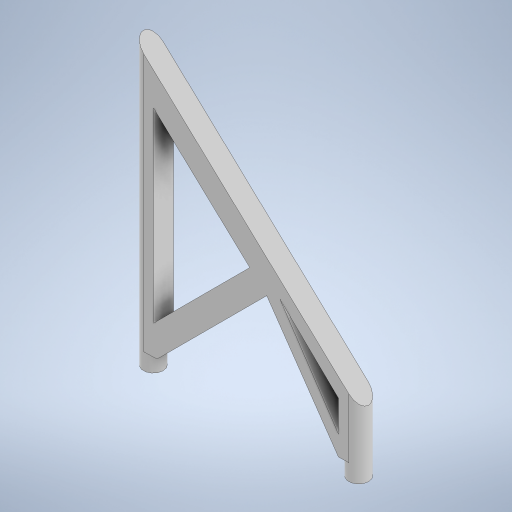
# Autodesk Inventor part: ControlPanel_Middle
Saved by Autodesk Inventor 2024 (Build 280153000, 153)
## iProperties
Created: 2024-04-17
Part Number: ControlPanel_Middle
Material: Generic
Document SubType Name: Modeling
Designer: ringl
Density: 1 g/cm^3
Appearance: Default
Author: ringl
Autodesk Inventor part; units mm, degrees
ref_plane "YZ Plane" through (0, 0, 0) normal (1, 0, 0) x (0, 1, 0)
ref_plane "XZ Plane" through (0, 0, 0) normal (0, 1, 0) x (-1, 0, 0)
sketch "Sketch1" plane through (0, 0, 0) normal (0, 1, 0) x (-1, 0, 0)
  circle A0 centre (0, 0) radius 1.5
  circle A1 centre (0, -51) radius 1.5
  circle A2 centre (30, -1) radius 1.5
  circle A3 centre (30, -50) radius 1.5
  dimension "d0" = 3
  dimension "d1" = 3
  dimension "d2" = 3
  dimension "d3" = 3
  dimension "d5" = 49
  dimension "d6" = 1
  dimension "d7" = 30
  dimension "d8" = 51
  constraints: 4 centre point, 2 vertical alignment, 1 coincident
  measures "d0" diameter of A0
  measures "d1" diameter of A1
  measures "d2" diameter of A2
  measures "d3" diameter of A3
  measures "d5" distance of A3.centre A2.centre
  measures "d6" vertical distance of point (0, 0) A2.centre
  measures "d7" horizontal distance of A2.centre point (0, 0)
  measures "d8" distance of point (0, 0) A1.centre
extrude "Extrusion1" add sketch "Sketch1" along normal blind 2.5
sketch "Sketch2" plane through (-30, 2.5, -1) normal (0, 1, 0) x (1, 0, 0)
  circle A0 centre (0, 0) radius 1.5 projected
  line L0 (0, -1.5) -> (30, -2.5)
  circle A1 centre (30, -1) radius 1.5 projected
  line L1 (30, 0.5) -> (0, 1.5)
  circle A2 centre (0, 49) radius 1.5 projected
  circle A3 centre (30, 50) radius 1.5 projected
  line L2 (0, 50.5) -> (29.95, 51.4992)
  line L3 (30, 48.5) -> (0.05, 47.5008)
  constraints: 8 end point, 8 point on circle, 5 vertical alignment, 2 tangent, 1 parallel
extrude "Extrusion2" add sketch "Sketch2" along normal blind 45
ref_plane "Work Plane1" through (0, 0, 2) normal (0, 0, 1) x (1, 0, 0)
sketch "Sketch3" plane through (0, 0, 2) normal (0, 0, 1) x (1, 0, 0)
  line L0 (1.5, 0) -> (1.5, 47.5) projected
  line L1 (1.5, 10) -> (-31.5, 43)
  line L2 (-31.5, 0) -> (-31.5, 47.5) projected
  line L3 (1.5, 0) -> (-1.5, 0) projected
  line L4 (-31.5, 43) -> (-31.5, 47.5)
  line L5 (-31.5, 0) -> (-31.5, 47.5) projected
  line L6 (1.5, 47.5) -> (1.5, 10)
  line L7 (1.5, 47.5) -> (-31.5, 47.5)
  line L8 (0, 2.5) -> (-29.9001, 2.5) projected
  line L9 (-1.5, 2.5) -> (-28, 2.5)
  line L10 (-28, 2.5) -> (-11.9749, 18.5251)
  line L11 (-11.9749, 18.5251) -> (-1.5, 2.5)
  line L12 (-28.5, 6.9497) -> (-14.4497, 21)
  line L13 (-14.4497, 21) -> (-28.5, 35.0503)
  line L14 (-31.5, 0) -> (-31.5, 47.5) projected
  line L15 (-10.0429, 18.9973) -> (-1.5, 5.5)
  line L16 (-1.5, 5.5) -> (-1.5, 10.1716)
  line L17 (-1.5, 10.1716) -> (-10.0429, 18.9973)
  line L18 (-28.5, 35.0503) -> (-28.5, 6.9497)
  point P0 (0, 0)
  point P1 (-15, 26.5)
  point P2 (-31.5, 38.0503)
  point P3 (-31.5, 3.9497)
  dimension "d14" = 45
  dimension "d15" = 10
  dimension "d18" = 3.5
  dimension "d19" = 3.5
  dimension "d20" = 3.5
  dimension "d21" = 3.5
  dimension "d22" = 45
  dimension "d23" = 3
  dimension "d24" = 1.8
  dimension "d25" = 3
  dimension "d26" = 2
  dimension "d27" = 12.2831
  dimension "d28" = 3
  constraints: 26 end point, 4 point on line, 2 collinear, 2 parallel, 2 vertical, 2 vertical alignment, 1 midpoint, 1 perpendicular
  measures "d14" angle of L3 L1
  measures "d15" distance of L0.start L1.start
  measures "d18" horizontal distance of L2.start L9.end
  measures "d19" distance from line of L1 L10.end
  measures "d20" distance from line of point (-15, 26.5) L13
  measures "d21" distance between parallel lines of L12 L10
  measures "d22" angle of L9 L10
  measures "d23" horizontal distance of L9.start L0.start
  measures "d24" distance from line of L15.start L1
  measures "d25" distance of L9.start L15.end
  measures "d26" distance from line of L1 L16.end
  measures "d27" distance of L16.end L15.start
  measures "d28" distance from line of L5 L12.start
extrude "Extrusion3" cut sketch "Sketch3" against normal through all
sketch "Sketch4" plane through (0, 0, 2) normal (0, 0, 1) x (1, 0, 0)
  line L0 (1.5, 0) -> (-1.5, 0) projected
  line L1 (-31.5, 0) -> (-31.5, 43) projected
  line L2 (1.5, 0) -> (-31.5, 0)
  line L3 (-31.5, 0) -> (-31.5, 43)
  line L4 (-31.5, 43) -> (1.5, 43)
  line L5 (1.5, 43) -> (1.5, 0)
  point P0 (0, 0)
  dimension "d29" = 43
  constraints: 8 end point, 2 parallel, 1 horizontal, 1 perpendicular, 1 point on line
  measures "d29" distance between parallel lines of L2 L4
extrude "Extrusion4" cut sketch "Sketch4" against normal blind 10
body "Solid1"
